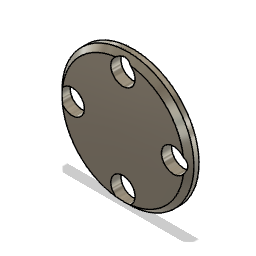
cryo contact clamp v3 (Autodesk Fusion 360 design; units mm, degrees)
Autodesk Fusion 360 part; units mm, degrees
note: some values were not read from the file. Set by a fixed rule: the direction of a hole.
sketch "Sketch1" plane through (0, 0, 0) normal (0, 0, 1) x (1, 0, 0)
  circle A0 centre (0, 0) radius 10 construction
  circle A1 centre (0, 0) radius 13
  point P0 (10, 0)
  point P1 (0, 10)
  point P2 (-10, 0)
  point P3 (0, -10)
  dimension "d1" = 20
  dimension "d2" = 26
  dimension "d4" = 360
  constraint coincident A0.centre A1.centre
  constraint coincident A0 P0
  constraint horizontal A0.centre P0
  measures "d1" diameter of A0
  measures "d2" diameter of A1
extrude "Extrude1" add sketch "Sketch1" along normal blind 2
hole "Hole1" at (-10, 0, 0) at (0, -10, 0) at (10, 0, 0) at (0, 10, 0) direction (0, 0, 1) diameter 4.8 depth 10 tip angle 118
chamfer "Chamfer1" distance 1 angle 45 1 edges at (-12.1203, -4.701, 2)
